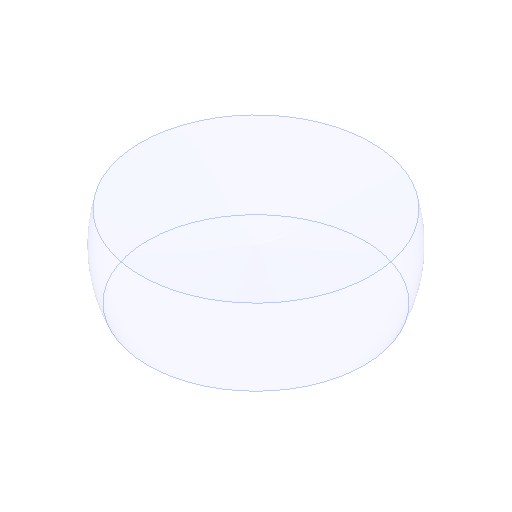
# Autodesk Inventor part: lidarFOV
Saved by Autodesk Inventor 2025 (Build 290162000, 162)
## iProperties
Created: 2024-11-19
Part Number: lidarFOV
Material: Generic
Document SubType Name: Modeling
Designer: derm
Density: 1 g/cm^3
Appearance: Clear - Blue
Author: derm
Autodesk Inventor part; units mm, degrees
ref_plane "YZ Plane" through (0, 0, 0) normal (1, 0, 0) x (0, 1, 0)
ref_plane "XZ Plane" through (0, 0, 0) normal (0, 1, 0) x (-1, 0, 0)
ref_plane "XY Plane" through (0, 0, 0) normal (0, 0, 1) x (1, 0, 0)
sketch "Sketch1" plane through (0, 0, 0) normal (0, 0, 1) x (1, 0, 0)
  line L0 (0, 0) -> (0, 737.5343)
  line L1 (0, 0) -> (965.9258, 258.819)
  line L2 (0, 0) -> (906.3078, -422.6183)
  arc A0 (906.3078, -422.6183) -> (965.9258, 258.819) centre (0, 0) ccw
  line L3 (0, 0) -> (723.3035, 0)
  dimension "d0" = 2000
  dimension "d1" = 15
  dimension "d2" = 25
  constraints: 8 end point, 2 point on circle, 1 centre point, 1 coincident, 1 horizontal, 1 vertical
  measures "d0" diameter of A0
  measures "d1" angle of L1 L3
  measures "d2" angle of L2 L3
revolve "Revolution1" add sketch "Sketch1" angle 360 about axis through (0, 0, 0) along (0, 1, 0)
body "Solid1"
